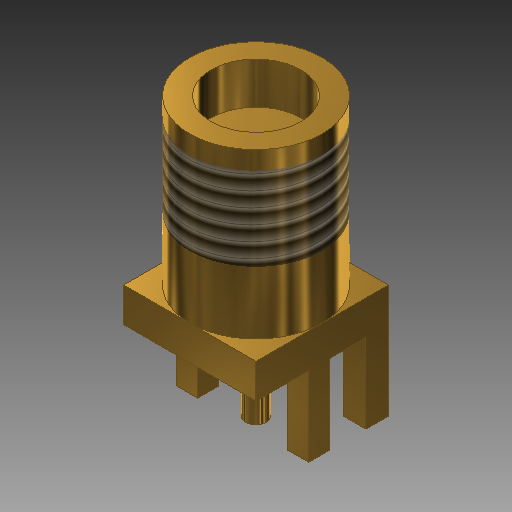
# Autodesk Inventor part: CON-SMA-EDGE-S
Saved by Autodesk Inventor 2019.1 (Build 231200000, 200)
## iProperties
Created: 2017-10-12
Part Number: CON-SMA-EDGE-S
Material: Messing, weicher Gelbton
Document SubType Name: Modeling
Designer: ryll
Density: 8.47 g/cm^3
Appearance: Messing - satiniert
Mass: 2.57459 g
Surface Area: 3.94246 cm^2
Volume: 0.303966 cm^3
Author: ryll
Autodesk Inventor part; units mm, degrees
ref_plane "YZ Plane" through (0, 0, 0) normal (1, 0, 0) x (0, 1, 0)
ref_plane "XZ Plane" through (0, 0, 0) normal (0, 1, 0) x (-1, 0, 0)
ref_plane "XY Plane" through (0, 0, 0) normal (0, 0, 1) x (1, 0, 0)
sketch "Skizze1" plane through (0, 0, 0) normal (0, 0, 1) x (1, 0, 0)
  line L0 (-3.175, -3.175) -> (3.175, -3.175)
  line L1 (3.175, -3.175) -> (3.175, 3.175)
  line L2 (3.175, 3.175) -> (-3.175, 3.175)
  line L3 (-3.175, 3.175) -> (-3.175, -3.175)
  line L4 (-3.175, -3.175) -> (3.175, 3.175) construction
  line L5 (3.175, -3.175) -> (-3.175, 3.175) construction
  point P0 (0, 0)
  dimension "d0" = 6.35
  dimension "d1" = 6.35
  constraints: 12 end point, 2 midpoint, 2 parallel, 1 horizontal, 1 perpendicular
  measures "d0" distance of L2.end L1.end
  measures "d1" distance of L1.end L0.end
extrude "Extrusion1" add sketch "Skizze1" along normal blind 1.65
sketch "Skizze2" plane through (0, 0, 1.65) normal (0, 0, 1) x (1, 0, 0)
  circle A0 centre (0, 0) radius 3.175
  dimension "d4" = 6.35
  constraints: 1 centre point, 1 coincident
  measures "d4" diameter of A0
extrude "Extrusion2" add sketch "Skizze2" along normal blind 7.87
sketch "Skizze3" plane through (0, 0, 9.52) normal (0, 0, 1) x (1, 0, 0)
  circle A0 centre (0, 0) radius 2.155
  dimension "d7" = 4.31
  constraints: 1 centre point, 1 coincident
  measures "d7" diameter of A0
extrude "Extrusion3" cut sketch "Skizze3" against normal blind 2
sketch "Skizze4" plane through (0, 0, 7.52) normal (0, 0, 1) x (1, 0, 0)
  circle A0 centre (0, 0) radius 0.38
  dimension "d10" = 0.76
  constraints: 1 centre point, 1 coincident
  measures "d10" diameter of A0
extrude "Extrusion4" cut sketch "Skizze4" against normal blind 5
thread "Gewinde1" size "1/4-36 UNS" class "2A" standard "ANSI Unified Screw Threads" length 4 offset 3
sketch "Skizze5" plane through (0, 0, 0) normal (0, 0, -1) x (-1, 0, 0)
  circle A0 centre (0, 0) radius 0.5
  dimension "d15" = 1
  constraints: 1 centre point, 1 coincident
  measures "d15" diameter of A0
extrude "Extrusion5" add sketch "Skizze5" along normal blind 3.81
sketch "Skizze6" plane through (0, 0, 0) normal (0, 0, -1) x (-1, 0, 0)
  line L0 (0, -4.445) -> (0, 4.445) projected
  line L1 (3.175, 3.175) -> (3.175, 0) projected
  arc A0 (-3.175, 0) -> (0, -3.175) centre (0, 0) ccw projected
  line L2 (3.175, 3.175) -> (2.105, 3.175)
  line L3 (2.105, 3.175) -> (2.105, 2.105)
  line L4 (2.105, 2.105) -> (3.175, 2.105)
  line L5 (3.175, 2.105) -> (3.175, 3.175)
  line L6 (-3.175, 3.175) -> (-2.105, 3.175)
  line L7 (-2.105, 3.175) -> (-2.105, 2.105)
  line L8 (-2.105, 2.105) -> (-3.175, 2.105)
  line L9 (-3.175, 2.105) -> (-3.175, 3.175)
  line L10 (-3.175, 3.175) -> (3.175, 3.175) projected
  line L11 (3.175, 0.375) -> (2.155, 0.375)
  line L12 (2.155, 0.375) -> (2.155, -0.645)
  line L13 (2.155, -0.645) -> (3.175, -0.645)
  line L14 (3.175, -0.645) -> (3.175, 0.375)
  line L15 (-3.175, -3.175) -> (-3.175, 3.175) projected
  line L16 (-3.175, 0.375) -> (-2.155, 0.375)
  line L17 (-2.155, 0.375) -> (-2.155, -0.645)
  line L18 (-2.155, -0.645) -> (-3.175, -0.645)
  line L19 (-3.175, -0.645) -> (-3.175, 0.375)
  dimension "d22" = 1.07
  dimension "d23" = 1.07
  dimension "d24" = 1.07
  dimension "d25" = 1.07
  dimension "d28" = 1.02
  dimension "d29" = 1.02
  dimension "d30" = 1.02
  dimension "d31" = 1.02
  dimension "d32" = 1.73
  constraints: 32 end point, 8 parallel, 4 horizontal, 4 perpendicular, 4 point on line, 3 collinear
  measures "d22" distance of L4.end L3.end
  measures "d23" distance of L3.end L2.end
  measures "d24" distance of L7.end L8.end
  measures "d25" distance of L6.end L7.end
  measures "d28" distance of L13.end L12.end
  measures "d29" distance of L12.end L11.end
  measures "d30" distance of L17.end L18.end
  measures "d31" distance of L16.end L17.end
  measures "d32" distance between parallel lines of L8 L16
extrude "Extrusion6" add sketch "Skizze6" along normal blind 3.81 contours L1 L14 L13 L12 L11 | L2 L1 L4 L3 | L18 L15 A0 | A0 L15 L16 L17 L18 | L7 L8 L9 L6
